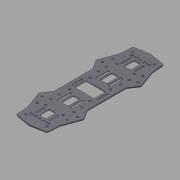
# Autodesk Inventor part: Bottom Plate
Saved by Autodesk Inventor 2011 SP2 (Build 150309200, 309)
## iProperties
Created: 2015-02-19
Part Number: Bottom Plate
Document SubType Name: Modeling
Designer: Greg Pavlik
Density: 1 g/cm^3
Author: Greg Pavlik
Autodesk Inventor part; units mm, degrees
ref_plane "YZ Plane" through (0, 0, 0) normal (1, 0, 0) x (0, 1, 0)
ref_plane "XZ Plane" through (0, 0, 0) normal (0, 1, 0) x (-1, 0, 0)
ref_plane "XY Plane" through (0, 0, 0) normal (0, 0, 1) x (1, 0, 0)
sketch "Sketch1" plane through (0, 0, 0) normal (0, 0, 1) x (1, 0, 0)
  line L0 (0, 92) -> (0, -92) construction
  line L1 (-25, 0) -> (25, 0) construction
  line L2 (-25, -28.8944) -> (-25, 28.8944)
  line L3 (-25.3359, 30.0038) -> (-33.4385, 42.1578)
  line L4 (-33.6538, 43.9512) -> (-24.5714, 68.9048)
  line L5 (-24.457, 69.4319) -> (-23.1215, 86.4007)
  line L6 (-21.475, 88.2134) -> (0, 92)
  line L7 (-25.3359, -30.0038) -> (-33.4385, -42.1578)
  line L8 (-33.6538, -43.9512) -> (-24.5714, -68.9048)
  line L9 (-24.457, -69.4319) -> (-23.1215, -86.4007)
  line L10 (-21.475, -88.2134) -> (0, -92)
  line L11 (25, -28.8944) -> (25, 28.8944)
  line L12 (25.3359, 30.0038) -> (33.4385, 42.1578)
  line L13 (33.6538, 43.9512) -> (24.5714, 68.9048)
  line L14 (24.457, 69.4319) -> (23.1215, 86.4007)
  line L15 (21.475, 88.2134) -> (0, 92)
  line L16 (25.3359, -30.0038) -> (33.4385, -42.1578)
  line L17 (33.6538, -43.9512) -> (24.5714, -68.9048)
  line L18 (24.457, -69.4319) -> (23.1215, -86.4007)
  line L19 (21.475, -88.2134) -> (0, -92)
  arc A0 (-33.6538, 43.9512) -> (-33.4385, 42.1578) centre (-31.7744, 43.2672) ccw
  arc A1 (-25, 28.8944) -> (-25.3359, 30.0038) centre (-27, 28.8944) ccw
  arc A2 (-25.3359, -30.0038) -> (-25, -28.8944) centre (-27, -28.8944) ccw
  arc A3 (-33.4385, -42.1578) -> (-33.6538, -43.9512) centre (-31.7744, -43.2672) ccw
  arc A4 (-24.457, -69.4319) -> (-24.5714, -68.9048) centre (-26.4508, -69.5889) ccw
  arc A5 (-23.1215, -86.4007) -> (-21.475, -88.2134) centre (-21.1277, -86.2438) ccw
  arc A6 (21.475, -88.2134) -> (23.1215, -86.4007) centre (21.1277, -86.2438) ccw
  arc A7 (24.5714, -68.9048) -> (24.457, -69.4319) centre (26.4508, -69.5889) ccw
  arc A8 (33.6538, -43.9512) -> (33.4385, -42.1578) centre (31.7744, -43.2672) ccw
  arc A9 (25, -28.8944) -> (25.3359, -30.0038) centre (27, -28.8944) ccw
  arc A10 (25.3359, 30.0038) -> (25, 28.8944) centre (27, 28.8944) ccw
  arc A11 (33.4385, 42.1578) -> (33.6538, 43.9512) centre (31.7744, 43.2672) ccw
  arc A12 (24.457, 69.4319) -> (24.5714, 68.9048) centre (26.4508, 69.5889) ccw
  arc A13 (-24.5714, 68.9048) -> (-24.457, 69.4319) centre (-26.4508, 69.5889) ccw
  arc A14 (-21.475, 88.2134) -> (-23.1215, 86.4007) centre (-21.1277, 86.2438) ccw
  arc A15 (23.1215, 86.4007) -> (21.475, 88.2134) centre (21.1277, 86.2438) ccw
  point P0 (0, 0)
  point P1 (-25, -29.5)
  point P2 (-25, 29.5)
  point P3 (-34, 43)
  point P4 (-24.4783, 69.1606)
  point P5 (-23, 87.9445)
  point P6 (-34, -43)
  point P7 (-24.4783, -69.1606)
  point P8 (-23, -87.9445)
  point P9 (25, -29.5)
  point P10 (25, 29.5)
  point P11 (34, 43)
  point P12 (24.4783, 69.1606)
  point P13 (23, 87.9445)
  point P14 (34, -43)
  point P15 (24.4783, -69.1606)
  point P16 (23, -87.9445)
  dimension "d0" = 46
  dimension "d1" = 160
  dimension "d2" = 184
  dimension "d3" = 50
  dimension "d4" = 68
  dimension "d5" = 86
  dimension "d6" = 59
  dimension "d7" = 104.5
  dimension "d8" = 164.5
  dimension "d9" = 2
  constraints: 40 end point, 32 point on circle, 32 point on line, 32 tangent, 16 centre point, 15 equal radius, 13 symmetric about line, 4 midpoint, 1 parallel, 1 perpendicular, 1 vertical
  measures "d0" distance of point (23, 87.944) point (-23, 87.944)
  measures "d1" angle of L15 L6
  measures "d2" distance of L0.end L0.start
  measures "d3" distance between parallel lines of L11 L2
  measures "d4" distance of point (34, 43) point (-34, 43)
  measures "d5" distance of point (-34, -43) point (-34, 43)
  measures "d6" distance of point (-25, -29.5) point (-25, 29.5)
  measures "d7" angle of L14 L15
  measures "d8" angle of L13 L14
  measures "d9" radius of A0
extrude "Extrusion1" add sketch "Sketch1" along normal mid plane 1.5
sketch "Sketch2" plane through (0, 0, 0.75) normal (0, 0, 1) x (1, 0, 0)
  line L0 (-25, -28.8944) -> (-25, 28.8944) construction
  line L1 (25, 28.8944) -> (25, -28.8944) construction
  line L2 (-25, 0) -> (25, 0) construction
  line L3 (0, 92) -> (0, -92) construction
  line L4 (-13.25, 8.75) -> (13.25, 8.75)
  line L5 (14.75, 7.25) -> (14.75, -7.25)
  line L6 (13.25, -8.75) -> (-13.25, -8.75)
  line L7 (-14.75, -7.25) -> (-14.75, 7.25)
  line L8 (-3, 38.25) -> (3, 38.25)
  line L9 (5, 36.25) -> (5, 22.25)
  line L10 (3, 20.25) -> (-3, 20.25)
  line L11 (-5, 22.25) -> (-5, 36.25)
  line L12 (-3, 71.25) -> (3, 71.25)
  line L13 (5, 69.25) -> (5, 58.25)
  line L14 (3, 56.25) -> (-3, 56.25)
  line L15 (-5, 58.25) -> (-5, 69.25)
  arc A0 (3, 56.25) -> (5, 58.25) centre (3, 58.25) ccw
  arc A1 (5, 36.25) -> (3, 38.25) centre (3, 36.25) ccw
  arc A2 (3, 20.25) -> (5, 22.25) centre (3, 22.25) ccw
  arc A3 (-5, 22.25) -> (-3, 20.25) centre (-3, 22.25) ccw
  arc A4 (-3, 38.25) -> (-5, 36.25) centre (-3, 36.25) ccw
  arc A5 (-5, 58.25) -> (-3, 56.25) centre (-3, 58.25) ccw
  arc A6 (-3, 71.25) -> (-5, 69.25) centre (-3, 69.25) ccw
  arc A7 (5, 69.25) -> (3, 71.25) centre (3, 69.25) ccw
  arc A8 (14.75, 7.25) -> (13.25, 8.75) centre (13.25, 7.25) ccw
  arc A9 (13.25, -8.75) -> (14.75, -7.25) centre (13.25, -7.25) ccw
  arc A10 (-14.75, -7.25) -> (-13.25, -8.75) centre (-13.25, -7.25) ccw
  arc A11 (-13.25, 8.75) -> (-14.75, 7.25) centre (-13.25, 7.25) ccw
  line L16 (-3, -38.25) -> (3, -38.25)
  line L17 (5, -36.25) -> (5, -22.25)
  line L18 (3, -20.25) -> (-3, -20.25)
  line L19 (-5, -22.25) -> (-5, -36.25)
  line L20 (-3, -71.25) -> (3, -71.25)
  line L21 (5, -69.25) -> (5, -58.25)
  line L22 (3, -56.25) -> (-3, -56.25)
  line L23 (-5, -58.25) -> (-5, -69.25)
  arc A12 (5, -58.25) -> (3, -56.25) centre (3, -58.25) ccw
  arc A13 (3, -38.25) -> (5, -36.25) centre (3, -36.25) ccw
  arc A14 (5, -22.25) -> (3, -20.25) centre (3, -22.25) ccw
  arc A15 (-3, -20.25) -> (-5, -22.25) centre (-3, -22.25) ccw
  arc A16 (-5, -36.25) -> (-3, -38.25) centre (-3, -36.25) ccw
  arc A17 (-3, -56.25) -> (-5, -58.25) centre (-3, -58.25) ccw
  arc A18 (-5, -69.25) -> (-3, -71.25) centre (-3, -69.25) ccw
  arc A19 (3, -71.25) -> (5, -69.25) centre (3, -69.25) ccw
  line L24 (11.2, -58.25) -> (11.2, -70.25)
  line L25 (9.2, -70.25) -> (9.2, -58.25)
  line L26 (11, -20.25) -> (11, -37.25)
  line L27 (8, -37.25) -> (8, -20.25)
  line L28 (20, 7) -> (20, -7)
  line L29 (18, -7) -> (18, 7)
  arc A20 (20, 7) -> (18, 7) centre (19, 7) ccw
  arc A21 (18, -7) -> (20, -7) centre (19, -7) ccw
  arc A22 (8, -37.25) -> (11, -37.25) centre (9.5, -37.25) ccw
  arc A23 (11, -20.25) -> (8, -20.25) centre (9.5, -20.25) ccw
  arc A24 (11.2, -58.25) -> (9.2, -58.25) centre (10.2, -58.25) ccw
  arc A25 (9.2, -70.25) -> (11.2, -70.25) centre (10.2, -70.25) ccw
  line L30 (11.2, 58.25) -> (11.2, 70.25)
  line L31 (9.2, 70.25) -> (9.2, 58.25)
  line L32 (11, 20.25) -> (11, 37.25)
  line L33 (8, 37.25) -> (8, 20.25)
  arc A26 (11, 37.25) -> (8, 37.25) centre (9.5, 37.25) ccw
  arc A27 (8, 20.25) -> (11, 20.25) centre (9.5, 20.25) ccw
  arc A28 (9.2, 58.25) -> (11.2, 58.25) centre (10.2, 58.25) ccw
  arc A29 (11.2, 70.25) -> (9.2, 70.25) centre (10.2, 70.25) ccw
  line L34 (-11.2, -58.25) -> (-11.2, -70.25)
  line L35 (-9.2, -70.25) -> (-9.2, -58.25)
  line L36 (-11, -20.25) -> (-11, -37.25)
  line L37 (-8, -37.25) -> (-8, -20.25)
  line L38 (-20, 7) -> (-20, -7)
  line L39 (-18, -7) -> (-18, 7)
  arc A30 (-18, 7) -> (-20, 7) centre (-19, 7) ccw
  arc A31 (-20, -7) -> (-18, -7) centre (-19, -7) ccw
  arc A32 (-11, -37.25) -> (-8, -37.25) centre (-9.5, -37.25) ccw
  arc A33 (-8, -20.25) -> (-11, -20.25) centre (-9.5, -20.25) ccw
  arc A34 (-9.2, -58.25) -> (-11.2, -58.25) centre (-10.2, -58.25) ccw
  arc A35 (-11.2, -70.25) -> (-9.2, -70.25) centre (-10.2, -70.25) ccw
  arc A36 (-11, 20.25) -> (-8, 20.25) centre (-9.5, 20.25) ccw
  line L40 (-11, 20.25) -> (-11, 37.25)
  line L41 (-8, 37.25) -> (-8, 20.25)
  arc A37 (-8, 37.25) -> (-11, 37.25) centre (-9.5, 37.25) ccw
  line L42 (-9.2, 70.25) -> (-9.2, 58.25)
  arc A38 (-11.2, 58.25) -> (-9.2, 58.25) centre (-10.2, 58.25) ccw
  line L43 (-11.2, 58.25) -> (-11.2, 70.25)
  arc A39 (-9.2, 70.25) -> (-11.2, 70.25) centre (-10.2, 70.25) ccw
  line L44 (6.5, -75) -> (12.5, -75)
  line L45 (14.5, -75) -> (14.5, -77)
  line L46 (12.5, -77) -> (6.5, -77)
  line L47 (4.5, -77) -> (4.5, -75)
  arc A40 (4.5, -77) -> (6.5, -77) centre (5.5, -77) ccw
  arc A41 (12.5, -77) -> (14.5, -77) centre (13.5, -77) ccw
  arc A42 (14.5, -75) -> (12.5, -75) centre (13.5, -75) ccw
  arc A43 (6.5, -75) -> (4.5, -75) centre (5.5, -75) ccw
  line L48 (-6.5, -75) -> (-12.5, -75)
  line L49 (-14.5, -75) -> (-14.5, -77)
  line L50 (-12.5, -77) -> (-6.5, -77)
  line L51 (-4.5, -77) -> (-4.5, -75)
  arc A44 (-6.5, -77) -> (-4.5, -77) centre (-5.5, -77) ccw
  arc A45 (-14.5, -77) -> (-12.5, -77) centre (-13.5, -77) ccw
  arc A46 (-12.5, -75) -> (-14.5, -75) centre (-13.5, -75) ccw
  arc A47 (-4.5, -75) -> (-6.5, -75) centre (-5.5, -75) ccw
  line L52 (6.5, 75) -> (12.5, 75)
  line L53 (14.5, 75) -> (14.5, 77)
  line L54 (12.5, 77) -> (6.5, 77)
  line L55 (4.5, 77) -> (4.5, 75)
  arc A48 (6.5, 77) -> (4.5, 77) centre (5.5, 77) ccw
  arc A49 (14.5, 77) -> (12.5, 77) centre (13.5, 77) ccw
  arc A50 (12.5, 75) -> (14.5, 75) centre (13.5, 75) ccw
  arc A51 (4.5, 75) -> (6.5, 75) centre (5.5, 75) ccw
  line L56 (-6.5, 75) -> (-12.5, 75)
  line L57 (-4.5, 77) -> (-4.5, 75)
  arc A52 (-4.5, 77) -> (-6.5, 77) centre (-5.5, 77) ccw
  line L58 (-12.5, 77) -> (-6.5, 77)
  arc A53 (-14.5, 75) -> (-12.5, 75) centre (-13.5, 75) ccw
  arc A54 (-12.5, 77) -> (-14.5, 77) centre (-13.5, 77) ccw
  line L59 (-14.5, 75) -> (-14.5, 77)
  arc A55 (-6.5, 75) -> (-4.5, 75) centre (-5.5, 75) ccw
  point P0 (0, 0)
  dimension "d12" = 2
  dimension "d13" = 1.5
  dimension "d14" = 29.5
  dimension "d15" = 17.5
  dimension "d16" = 11.5
  dimension "d17" = 18
  dimension "d18" = 18
  dimension "d19" = 15
  dimension "d20" = 10
  dimension "d21" = 1
  dimension "d22" = 1.5
  dimension "d23" = 1
  dimension "d24" = 38
  dimension "d25" = 14
  dimension "d26" = 13.25
  dimension "d27" = 17
  dimension "d28" = 19
  dimension "d29" = 20.4
  dimension "d30" = 12
  dimension "d31" = 21
  dimension "d35" = 10
  dimension "d36" = 2
  dimension "d37" = 1
  dimension "d38" = 4.5
  dimension "d39" = 15
  constraints: 116 end point, 112 point on circle, 102 symmetric about line, 56 centre point, 40 tangent, 16 point on line, 13 equal radius, 13 parallel, 5 perpendicular, 4 horizontal, 2 midpoint, 1 collinear, 39 other
  measures "d12" radius of A0
  measures "d13" radius of A8
  measures "d14" distance between parallel lines of L5 L7
  measures "d15" distance between parallel lines of L6 L4
  measures "d16" distance between parallel lines of L10 L4
  measures "d17" distance between parallel lines of L8 L10
  measures "d18" distance between parallel lines of L14 L8
  measures "d19" distance between parallel lines of L12 L14
  measures "d20" distance between parallel lines of L13 L15
  measures "d21" radius of A25
  measures "d22" radius of A22
  measures "d23" radius of A21
  measures "d24" distance of A31.centre A21.centre
  measures "d25" distance of A21.centre A20.centre
  measures "d26" vertical distance of A31.centre A33.centre
  measures "d27" distance of A32.centre A33.centre
  measures "d28" distance of A23.centre A33.centre
  measures "d29" distance of A24.centre A34.centre
  measures "d30" distance of A35.centre A34.centre
  measures "d31" vertical distance of A34.centre A32.centre
  measures "d35" distance between parallel lines of L45 L47
  measures "d36" distance between parallel lines of L46 L44
  measures "d37" radius of A41
  measures "d38" distance between parallel lines of L47 L3
  measures "d39" distance from line of L3.end L46
extrude "Extrusion2" cut sketch "Sketch2" against normal through all
sketch "Sketch3" plane through (0, 0, 0.75) normal (0, 0, 1) x (1, 0, 0)
  line L0 (-25, -28.8944) -> (-25, 28.8944) construction
  line L1 (25, 28.8944) -> (25, -28.8944) construction
  line L2 (-25, 0) -> (25, 0) construction
  line L3 (0, 92) -> (0, -92) construction
  line L4 (33.6538, -43.9512) -> (24.5714, -68.9048) construction
  line L5 (26.7414, -45.4) -> (22.4662, -57.1462) construction
  line L6 (22.4662, -57.1462) -> (13.0692, -53.726) construction
  line L7 (13.0692, -53.726) -> (17.3445, -41.9798) construction
  line L8 (17.3445, -41.9798) -> (26.7414, -45.4) construction
  point P0 (0, 0)
  point P1 (-17, 29.5)
  point P2 (-15.25, 15.25)
  point P3 (17, 29.5)
  point P4 (15.25, 15.25)
  point P5 (-17, -29.5)
  point P6 (-15.25, -15.25)
  point P7 (15.25, -15.25)
  point P8 (17, -29.5)
  point P9 (-16, 81)
  point P10 (0, 76)
  point P11 (16, 81)
  point P12 (-16, -81)
  point P13 (0, -76)
  point P14 (16, -81)
  point P15 (-26.7414, -45.4)
  point P16 (-17.3445, -41.9798)
  point P17 (-13.0692, -53.726)
  point P18 (-22.4662, -57.1462)
  point P19 (26.7414, 45.4)
  point P20 (17.3445, 41.9798)
  point P21 (13.0692, 53.726)
  point P22 (22.4662, 57.1462)
  point P23 (-13.0692, 53.726)
  point P24 (-17.3445, 41.9798)
  point P25 (-26.7414, 45.4)
  point P26 (-22.4662, 57.1462)
  dimension "d42" = 30.5
  dimension "d43" = 30.5
  dimension "d44" = 34
  dimension "d45" = 59
  dimension "d46" = 32
  dimension "d47" = 5
  dimension "d48" = 162
  dimension "d49" = 12.5
  dimension "d50" = 6
  dimension "d51" = 10
  dimension "d52" = 45.4
  constraints: 22 symmetric about line, 12 end point, 4 coincident, 3 parallel, 2 midpoint, 2 perpendicular, 1 point on line
  measures "d42" distance of point (-15.25, -15.25) point (-15.25, 15.25)
  measures "d43" distance of point (15.25, 15.25) point (-15.25, 15.25)
  measures "d44" distance of point (17, 29.5) point (-17, 29.5)
  measures "d45" distance of point (-17, -29.5) point (-17, 29.5)
  measures "d46" distance of point (16, 81) point (-16, 81)
  measures "d47" vertical distance of point (0, 76) point (16, 81)
  measures "d48" distance of point (16, 81) point (16, -81)
  measures "d49" distance between parallel lines of L6 L8
  measures "d50" distance between parallel lines of L4 L5
  measures "d51" distance between parallel lines of L7 L5
  measures "d52" distance from line of L2 point (26.741, -45.4)
hole "Hole1" at (-17, 29.5, 0.75) at (-15.25, 15.25, 0.75) at (15.25, 15.25, 0.75) at (17, 29.5, 0.75) at (-17, -29.5, 0.75) at (-15.25, -15.25, 0.75) at (15.25, -15.25, 0.75) at (17, -29.5, 0.75) at (-16, 81, 0.75) at (0, 76, 0.75) at (16, 81, 0.75) at (-16, -81, 0.75) at (0, -76, 0.75) at (16, -81, 0.75) at (26.7414, -45.4, 0.75) at (17.3445, -41.9798, 0.75) at (13.0692, -53.726, 0.75) at (22.4662, -57.1462, 0.75) at (-13.0692, -53.726, 0.75) at (-17.3445, -41.9798, 0.75) at (-26.7414, -45.4, 0.75) at (-22.4662, -57.1462, 0.75) at (-13.0692, 53.726, 0.75) at (-17.3445, 41.9798, 0.75) at (-26.7414, 45.4, 0.75) at (-22.4662, 57.1462, 0.75) at (13.0692, 53.726, 0.75) at (17.3445, 41.9798, 0.75) at (26.7414, 45.4, 0.75) at (22.4662, 57.1462, 0.75) direction (0, 0, -1) diameter 3 end through all
chamfer "Chamfer1" distance 0.15 angle 45 60 edges at (-16, -79.5, 0.75) (-22.4662, -55.6462, 0.75) (-26.7414, -43.9, 0.75) (-17.3445, -40.4798, 0.75) (-13.0692, -52.226, 0.75) (-17, -28, 0.75) (-15.25, -13.75, 0.75) (0, -74.5, 0.75) (13.0692, -52.226, 0.75) (16, -79.5, 0.75) (17.3445, -40.4798, 0.75) (22.4662, -55.6462, 0.75) (26.7414, -43.9, 0.75) (17, -28, 0.75) (15.25, -13.75, 0.75) (-15.25, 16.75, 0.75) (-17, 31, 0.75) (-26.7414, 46.9, 0.75) (-22.4662, 58.6462, 0.75) (-17.3445, 43.4798, 0.75) (-16, 82.5, 0.75) (-13.0692, 55.226, 0.75) (0, 77.5, 0.75) (15.25, 16.75, 0.75) (17, 31, 0.75) (13.0692, 55.226, 0.75) (17.3445, 43.4798, 0.75) (26.7414, 46.9, 0.75) (22.4662, 58.6462, 0.75) (16, 82.5, 0.75) (-16, -79.5, -0.75) (-22.4662, -55.6462, -0.75) (-26.7414, -43.9, -0.75) (-17.3445, -40.4798, -0.75) (-13.0692, -52.226, -0.75) (-17, -28, -0.75) (-15.25, -13.75, -0.75) (0, -74.5, -0.75) (13.0692, -52.226, -0.75) (16, -79.5, -0.75) (17.3445, -40.4798, -0.75) (22.4662, -55.6462, -0.75) (26.7414, -43.9, -0.75) (17, -28, -0.75) (15.25, -13.75, -0.75) (-15.25, 16.75, -0.75) (-17, 31, -0.75) (-26.7414, 46.9, -0.75) (-22.4662, 58.6462, -0.75) (-17.3445, 43.4798, -0.75) (-16, 82.5, -0.75) (-13.0692, 55.226, -0.75) (0, 77.5, -0.75) (15.25, 16.75, -0.75) (17, 31, -0.75) (13.0692, 55.226, -0.75) (17.3445, 43.4798, -0.75) (26.7414, 46.9, -0.75) (22.4662, 58.6462, -0.75) (16, 82.5, -0.75)
chamfer "Chamfer2" distance 0.15 angle 45 160 edges at (-14.75, 0, -0.75) (-14.3107, -8.3107, -0.75) (0, -8.75, -0.75) (14.3107, -8.3107, -0.75) (14.75, 0, -0.75) (14.3107, 8.3107, -0.75) (0, 8.75, -0.75) (-14.3107, 8.3107, -0.75) (-14.75, 0, 0.75) (-14.3107, 8.3107, 0.75) (0, 8.75, 0.75) (14.3107, 8.3107, 0.75) (14.75, 0, 0.75) (14.3107, -8.3107, 0.75) (0, -8.75, 0.75) (-14.3107, -8.3107, 0.75) (-18, 0, 0.75) (-19, -8, 0.75) (-20, 0, 0.75) (-19, 8, 0.75) (-18, 0, -0.75) (-19, 8, -0.75) (-20, 0, -0.75) (-19, -8, -0.75) (-9.5, -18.75, 0.75) (-8, -28.75, 0.75) (-9.5, -38.75, 0.75) (-11, -28.75, 0.75) (-4.4142, -20.8358, -0.75) (-5, -29.25, -0.75) (-4.4142, -37.6642, -0.75) (0, -38.25, -0.75) (4.4142, -37.6642, -0.75) (5, -29.25, -0.75) (4.4142, -20.8358, -0.75) (0, -20.25, -0.75) (-4.4142, -20.8358, 0.75) (0, -20.25, 0.75) (4.4142, -20.8358, 0.75) (5, -29.25, 0.75) (4.4142, -37.6642, 0.75) (0, -38.25, 0.75) (-4.4142, -37.6642, 0.75) (-5, -29.25, 0.75) (-9.5, -18.75, -0.75) (-11, -28.75, -0.75) (-9.5, -38.75, -0.75) (-8, -28.75, -0.75) (9.5, -18.75, 0.75) (11, -28.75, 0.75) (9.5, -38.75, 0.75) (8, -28.75, 0.75) (9.5, -18.75, -0.75) (8, -28.75, -0.75) (9.5, -38.75, -0.75) (11, -28.75, -0.75) (0, 38.25, -0.75) (-4.4142, 37.6642, -0.75) (-5, 29.25, -0.75) (-4.4142, 20.8358, -0.75) (0, 20.25, -0.75) (4.4142, 20.8358, -0.75) (5, 29.25, -0.75) (4.4142, 37.6642, -0.75) (-9.5, 18.75, 0.75) (-11, 28.75, 0.75) (-9.5, 38.75, 0.75) (-8, 28.75, 0.75) (8, 28.75, 0.75) (9.5, 38.75, 0.75) (11, 28.75, 0.75) (9.5, 18.75, 0.75) (0, 38.25, 0.75) (4.4142, 37.6642, 0.75) (5, 29.25, 0.75) (4.4142, 20.8358, 0.75) (0, 20.25, 0.75) (-4.4142, 20.8358, 0.75) (-5, 29.25, 0.75) (-4.4142, 37.6642, 0.75) (20, 0, 0.75) (19, -8, 0.75) (18, 0, 0.75) (19, 8, 0.75) (18, 0, -0.75) (19, -8, -0.75) (20, 0, -0.75) (19, 8, -0.75) (-9.2, -64.25, 0.75) (-10.2, -71.25, 0.75) (-11.2, -64.25, 0.75) (-10.2, -57.25, 0.75) (-11.2, -64.25, -0.75) (-10.2, -71.25, -0.75) (-9.2, -64.25, -0.75) (-10.2, -57.25, -0.75) (-5, -63.75, -0.75) (-4.4142, -70.6642, -0.75) (0, -71.25, -0.75) (4.4142, -70.6642, -0.75) (5, -63.75, -0.75) (4.4142, -56.8358, -0.75) (0, -56.25, -0.75) (-4.4142, -56.8358, -0.75) (-5, -63.75, 0.75) (-4.4142, -56.8358, 0.75) (0, -56.25, 0.75) (4.4142, -56.8358, 0.75) (5, -63.75, 0.75) (4.4142, -70.6642, 0.75) (0, -71.25, 0.75) (-4.4142, -70.6642, 0.75) (11.2, -64.25, -0.75) (10.2, -57.25, -0.75) (9.2, -64.25, -0.75) (10.2, -71.25, -0.75) (9.2, -64.25, 0.75) (10.2, -57.25, 0.75) (11.2, -64.25, 0.75) (10.2, -71.25, 0.75) (-5, 63.75, -0.75) (-4.4142, 56.8358, -0.75) (0, 56.25, -0.75) (4.4142, 56.8358, -0.75) (5, 63.75, -0.75) (4.4142, 70.6642, -0.75) (0, 71.25, -0.75) (-4.4142, 70.6642, -0.75) (-5, 63.75, 0.75) (-4.4142, 70.6642, 0.75) (0, 71.25, 0.75) (4.4142, 70.6642, 0.75) (5, 63.75, 0.75) (4.4142, 56.8358, 0.75) (0, 56.25, 0.75) (-4.4142, 56.8358, 0.75) (-9.2, 64.25, -0.75) (-10.2, 71.25, -0.75) (-11.2, 64.25, -0.75) (-10.2, 57.25, -0.75) (-11.2, 64.25, 0.75) (-10.2, 71.25, 0.75) (-9.2, 64.25, 0.75) (-10.2, 57.25, 0.75) (8, 28.75, -0.75) (9.5, 18.75, -0.75) (11, 28.75, -0.75) (9.5, 38.75, -0.75) (11.2, 64.25, 0.75) (10.2, 57.25, 0.75) (9.2, 64.25, 0.75) (10.2, 71.25, 0.75) (-8, 28.75, -0.75) (-9.5, 38.75, -0.75) (-11, 28.75, -0.75) (-9.5, 18.75, -0.75) (9.2, 64.25, -0.75) (10.2, 57.25, -0.75) (11.2, 64.25, -0.75) (10.2, 71.25, -0.75)
chamfer "Chamfer3" distance 0.1 angle 45 61 edges at (-9.5, 75, -0.75) (-9.5, 75, 0.75) (-13.5, 74, 0.75) (-14.5, 76, 0.75) (-13.5, 78, 0.75) (-9.5, 77, 0.75) (-9.5, 77, -0.75) (-5.5, 78, 0.75) (-4.5, 76, 0.75) (-5.5, 74, 0.75) (-5.5, 78, -0.75) (-4.5, 76, -0.75) (-5.5, 74, -0.75) (5.5, 78, 0.75) (4.5, 76, 0.75) (5.5, 74, 0.75) (5.5, 74, -0.75) (4.5, 76, -0.75) (5.5, 78, -0.75) (9.5, 75, -0.75) (9.5, 75, 0.75) (13.5, 78, 0.75) (14.5, 76, 0.75) (13.5, 74, 0.75) (9.5, 77, 0.75) (9.5, 77, -0.75) (14.5, 76, -0.75) (13.5, 78, -0.75) (13.5, 74, -0.75) (9.5, -77, 0.75) (9.5, -77, -0.75) (9.5, -75, 0.75) (9.5, -75, -0.75) (4.5, -76, -0.75) (5.5, -78, -0.75) (5.5, -74, -0.75) (4.5, -76, 0.75) (5.5, -74, 0.75) (5.5, -78, 0.75) (13.5, -78, 0.75) (14.5, -76, 0.75) (13.5, -74, 0.75) (14.5, -76, -0.75) (13.5, -74, -0.75) (13.5, -78, -0.75) (-14.5, -76, 0.75) (-13.5, -74, 0.75) (-13.5, -78, 0.75) (-13.5, -78, -0.75) (-14.5, -76, -0.75) (-13.5, -74, -0.75) (-5.5, -78, 0.75) (-4.5, -76, 0.75) (-5.5, -74, 0.75) (-5.5, -78, -0.75) (-4.5, -76, -0.75) (-5.5, -74, -0.75) (-9.5, -77, -0.75) (-9.5, -77, 0.75) (-9.5, -75, 0.75) (-9.5, -75, -0.75)
chamfer "Chamfer4" distance 0.15 angle 45 68 edges at (-29.3872, -36.0808, 0.75) (-25.0858, -29.474, 0.75) (-25, 0, 0.75) (-25.0858, 29.474, 0.75) (-29.3872, 36.0808, 0.75) (-33.7602, 43.0288, 0.75) (-29.1126, 56.428, 0.75) (-24.4963, 69.1645, 0.75) (-23.7892, 77.9163, 0.75) (-22.6081, 87.5885, 0.75) (-10.7375, 90.1067, 0.75) (-33.7602, -43.0288, 0.75) (-29.1126, -56.428, 0.75) (-24.4963, -69.1645, 0.75) (-23.7892, -77.9163, 0.75) (-22.6081, -87.5885, 0.75) (-10.7375, -90.1067, 0.75) (10.7375, -90.1067, -0.75) (22.6081, -87.5885, -0.75) (23.7892, -77.9163, -0.75) (24.4963, -69.1645, -0.75) (29.1126, -56.428, -0.75) (33.7602, -43.0288, -0.75) (29.3872, -36.0808, -0.75) (25.0858, -29.474, -0.75) (25, 0, -0.75) (25.0858, 29.474, -0.75) (29.3872, 36.0808, -0.75) (33.7602, 43.0288, -0.75) (29.1126, 56.428, -0.75) (24.4963, 69.1645, -0.75) (23.7892, 77.9163, -0.75) (22.6081, 87.5885, -0.75) (10.7375, 90.1067, -0.75) (10.7375, -90.1067, 0.75) (22.6081, -87.5885, 0.75) (23.7892, -77.9163, 0.75) (24.4963, -69.1645, 0.75) (29.1126, -56.428, 0.75) (33.7602, -43.0288, 0.75) (29.3872, -36.0808, 0.75) (25.0858, -29.474, 0.75) (25, 0, 0.75) (25.0858, 29.474, 0.75) (29.3872, 36.0808, 0.75) (33.7602, 43.0288, 0.75) (29.1126, 56.428, 0.75) (24.4963, 69.1645, 0.75) (23.7892, 77.9163, 0.75) (22.6081, 87.5885, 0.75) (10.7375, 90.1067, 0.75) (-10.7375, -90.1067, -0.75) (-22.6081, -87.5885, -0.75) (-23.7892, -77.9163, -0.75) (-24.4963, -69.1645, -0.75) (-29.1126, -56.428, -0.75) (-33.7602, -43.0288, -0.75) (-29.3872, -36.0808, -0.75) (-25.0858, -29.474, -0.75) (-25, 0, -0.75) (-25.0858, 29.474, -0.75) (-29.3872, 36.0808, -0.75) (-33.7602, 43.0288, -0.75) (-29.1126, 56.428, -0.75) (-24.4963, 69.1645, -0.75) (-23.7892, 77.9163, -0.75) (-22.6081, 87.5885, -0.75) (-10.7375, 90.1067, -0.75)
body "Solid1"
